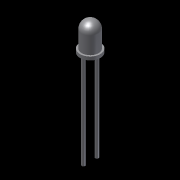
# Autodesk Inventor part: LED´s
Saved by Autodesk Inventor 2011 SP1 (Build 150282100, 282)
## iProperties
Created: 2012-07-13
Part Number: LED´s
Document SubType Name: Modeling
Designer: nfischer
Density: 1 g/cm^3
Author: nfischer
Autodesk Inventor part; units mm, degrees
ref_plane "YZ Plane" through (0, 0, 0) normal (1, 0, 0) x (0, 1, 0)
ref_plane "XZ Plane" through (0, 0, 0) normal (0, 1, 0) x (-1, 0, 0)
ref_plane "XY Plane" through (0, 0, 0) normal (0, 0, 1) x (1, 0, 0)
sketch "Skizze1" plane through (0, 0, 0) normal (0, 0, 1) x (1, 0, 0)
  circle A0 centre (0, 0) radius 2.5
  dimension "d0" = 5
  constraints: 1 centre point, 1 coincident
  measures "d0" diameter of A0
extrude "Extrusion1" add sketch "Skizze1" along normal blind 8.5
fillet "Rundung1" radius 2.5 1 edges at (-2.5, 0, 8.5)
sketch "Skizze2" plane through (0, 0, 0) normal (0, 0, -1) x (-1, 0, 0)
  circle A0 centre (0, 0) radius 2.5 projected
  circle A1 centre (0, 0) radius 3
  dimension "d4" = 6
  constraints: 1 centre point, 1 coincident
  measures "d4" diameter of A1
extrude "Extrusion2" add sketch "Skizze2" against normal blind 1
sketch "Skizze3" plane through (0, 0, 0) normal (0, 0, -1) x (-1, 0, 0)
  circle A0 centre (0, 0) radius 3 projected
  circle A1 centre (0, 2) radius 0.5
  circle A2 centre (0, -2) radius 0.5
  point P0 (0, 3)
  point P1 (0, -3)
  dimension "d7" = 1
  dimension "d8" = 1
  dimension "d9" = 1
  dimension "d10" = 1
  constraints: 2 centre point, 2 coincident, 2 point on circle
  measures "d7" distance of point (0, 2) A0.start
  measures "d8" distance of A0.end point (0, -2)
  measures "d9" diameter of A2
  measures "d10" diameter of A1
extrude "Extrusion3" add sketch "Skizze3" along normal blind 28 contours A1 | A2
